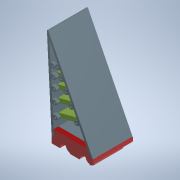
# Autodesk Inventor part: FingerEnclosure
Saved by Autodesk Inventor 2021 (Build 250183000, 183)
## iProperties
Created: 2020-03-10
Part Number: FingerEnclosure
Material: Generisch
Document SubType Name: Modeling
Designer: JochenAlt
Density: 1 g/cm^3
Appearance: Rot
Author: JochenAlt
Autodesk Inventor part; units mm, degrees
note: some values were not read from the file. Left out: dimensions or parameters whose unit could not be read.
ref_plane "YZ Plane" through (0, 0, 0) normal (1, 0, 0) x (0, 1, 0)
ref_plane "XZ Plane" through (0, 0, 0) normal (0, 1, 0) x (-1, 0, 0)
ref_plane "XY Plane" through (0, 0, 0) normal (0, 0, 1) x (1, 0, 0)
sketch "MainConstruction" plane through (0, 0, 0) normal (0, 0, 1) x (1, 0, 0)
  line L0 (-44.4573, 0) -> (45.9096, 0) construction
  line L1 (0, -41.3) -> (0, 41.3) construction
  line L2 (-12, 16.3923) -> (12, 16.3923) construction
  line L3 (6, -16.3923) -> (6, -10.3923) construction
  line L4 (6, -10.3923) -> (11.1962, -13.3923) construction
  line L5 (8.1962, -18.5885) -> (11.1962, -13.3923) construction
  line L6 (0, -16.3923) -> (6, -16.3923) construction
  line L7 (-6, -10.3923) -> (-6, -16.3923) construction
  line L8 (-6, -10.3923) -> (-11.1962, -13.3923) construction
  line L9 (0, 16.3923) -> (0, 0) construction
  line L10 (0, 0) -> (0, -16.3923) construction
  line L11 (-12, 14.3923) -> (12, 14.3923) construction
  line L12 (-12, 16.3923) -> (-12, 14.3923) construction
  line L13 (-12, 27) -> (12, 27) construction
  line L14 (-29.3827, -3.1077) -> (-17.3827, -23.8923) construction
  line L15 (0, 16.3923) -> (0, 27) construction
  line L16 (-23.3827, -13.5) -> (-14.1962, -8.1962) construction
  arc A0 (-2.6277, -14.0839) -> (-3.3698, -6.14) centre (-6, -10.3923) ccw construction
  arc A1 (3.3698, -6.14) -> (2.6277, -14.0839) centre (6, -10.3923) ccw construction
  line L17 (-27.2176, -1.8577) -> (-31.5477, -4.3577) construction
  line L18 (-15.2176, -22.6423) -> (-19.5477, -25.1423) construction
  line L19 (19.5477, -25.1423) -> (15.2176, -22.6423) construction
  circle A2 centre (0, 0) radius 22 construction
  line L20 (12, 14.3923) -> (12, 16.3923) construction
  line L21 (23.3827, -13.5) -> (14.1962, -8.1962) construction
  line L22 (20.1962, 2.1962) -> (14.1962, -8.1962) construction
  line L23 (11.1962, -13.3923) -> (14.1962, -8.1962) construction
  line L24 (-6, -16.3923) -> (0, -16.3923) construction
  line L25 (8.1962, -18.5885) -> (15.2176, -22.6423) construction
  line L26 (-15.2176, -22.6423) -> (-8.1962, -18.5885) construction
  line L27 (-12, 29.5) -> (-12, 24.5) construction
  line L28 (12, 29.5) -> (12, 24.5) construction
  line L29 (12, 24.5) -> (12, 16.3923) construction
  line L30 (-12, 24.5) -> (-12, 16.3923) construction
  line L31 (-11.1962, -13.3923) -> (-8.1962, -18.5885) construction
  line L32 (-11.1962, -13.3923) -> (-20.1962, 2.1962) construction
  line L33 (27.2176, -1.8577) -> (31.5477, -4.3577) construction
  line L34 (17.3827, -23.8923) -> (29.3827, -3.1077) construction
  line L35 (27.2176, -1.8577) -> (21.9687, 1.1728) construction
  line L36 (-27.2176, -1.8577) -> (-21.9687, 1.1728) construction
  line L37 (20.1962, 2.1962) -> (21.9687, 1.1728) construction
  line L38 (-21.9687, 1.1728) -> (-20.1962, 2.1962) construction
  line L39 (0, -16.3923) -> (0, -24.5) construction
  line L40 (0, -24.5) -> (0, -29.5) construction
  line L41 (0, -27) -> (24, -27) construction
  line L42 (18.4641, 3.1962) -> (6.4641, -17.5885) construction
  line L43 (-18.4641, 3.1962) -> (-6.4641, -17.5885) construction
  line L44 (-20.1962, 2.1962) -> (-18.4641, 3.1962) construction
  line L45 (20.1962, 2.1962) -> (18.4641, 3.1962) construction
  line L46 (3.3698, -6.14) -> (18.4641, 3.1962) construction
  line L47 (-18.4641, 3.1962) -> (-3.3698, -6.14) construction
  circle A3 centre (30.5, 27) radius 2.5 construction
  line L48 (12, 14.3923) -> (16.25, 14.3923) construction
  line L49 (16.25, 14.3923) -> (31.8962, 24.9262) construction
  line L50 (29.1038, 29.0738) -> (10.2677, 16.3923) construction
  line L51 (12, 16.3923) -> (10.2677, 16.3923) construction
  line L52 (8.1962, -18.5885) -> (6.4641, -17.5885) construction
  line L53 (6.4641, -17.5885) -> (2.6277, -14.0839) construction
  line L54 (-8.1962, -18.5885) -> (-6.4641, -17.5885) construction
  line L55 (-6.4641, -17.5885) -> (-2.6277, -14.0839) construction
sketch "Main" plane through (0, 0, 0) normal (0, 0, 1) x (1, 0, 0)
  line L0 (-20, 4) -> (-22.8714, 57.5994)
  line L1 (-23, 60) -> (-21.9249, 57.8498) construction
  line L2 (5, 4) -> (-20, 4)
  line L3 (-13.061, 37.1034) -> (-12.502, 35.9853)
  line L4 (-19.1427, 13.2337) -> (-18.7552, 6)
  line L5 (-19.7847, 25.2166) -> (-19.552, 20.8727) construction
  line L6 (-19.9203, 27.7479) -> (-19.6857, 23.3691)
  line L7 (-6.6518, 24.2849) -> (-4.3486, 19.6786)
  line L8 (-9.7309, 30.443) -> (-7.7698, 26.521)
  line L9 (-21.3047, 53.5907) -> (-16.1141, 43.2095)
  line L10 (-12.502, 35.9853) -> (-10.8489, 32.6791)
  line L11 (-21.3047, 53.5907) -> (-20.6838, 42.0008)
  line L12 (-20.2518, 33.9355) -> (-20.054, 30.2443)
  line L13 (-3.7896, 18.5606) -> (-3.2306, 17.4425)
  line L14 (-4.3486, 19.6786) -> (-3.7896, 18.5606)
  line L15 (-3.2306, 17.4425) -> (2.4907, 6) construction
  line L16 (-19.2765, 15.7301) -> (-19.7847, 25.2166) construction
  line L17 (-19.2096, 14.4819) -> (-19.2765, 15.7301)
  line L18 (-19.1427, 13.2337) -> (-19.2096, 14.4819)
  line L19 (-7.7698, 26.521) -> (-7.2108, 25.4029)
  line L20 (-7.2108, 25.4029) -> (-6.6518, 24.2849)
  line L21 (-6.6518, 24.2849) -> (-4.3486, 19.6786) construction
  line L22 (-19.7847, 25.2166) -> (-19.552, 20.8727)
  line L23 (-20.054, 30.2443) -> (-20.2518, 33.9355) construction
  line L24 (-19.9871, 28.9961) -> (-20.054, 30.2443)
  line L25 (-19.9203, 27.7479) -> (-19.9871, 28.9961)
  line L26 (-10.8489, 32.6791) -> (-10.2899, 31.5611)
  line L27 (-10.2899, 31.5611) -> (-9.7309, 30.443)
  line L28 (-9.7309, 30.443) -> (-7.7698, 26.521) construction
  line L29 (-20.3855, 36.4319) -> (-20.3186, 35.1837)
  line L30 (-13.6201, 38.2214) -> (-13.061, 37.1034)
  line L31 (-12.502, 35.9853) -> (-10.8489, 32.6791) construction
  line L32 (-20.2518, 33.9355) -> (-20.3186, 35.1837)
  line L33 (-18.7552, 6) -> (-19.1427, 13.2337) construction
  line L34 (-3.2306, 17.4425) -> (2.4907, 6)
  line L35 (-18.7552, 6) -> (2.4907, 6)
  arc A0 (-21.9249, 57.8498) -> (-22.8714, 57.5994) centre (-22.3721, 57.6262) ccw
  line L36 (-18.7552, 6) -> (-18.6481, 4)
  line L37 (2.4907, 6) -> (3.4907, 4)
  circle A1 centre (-12, 0) radius 1.05
  arc A2 (-14.9041, -0.7524) -> (-9, 0) centre (-12, 0) ccw
  circle A3 centre (0, 0) radius 1.05
  arc A4 (-3, 0) -> (3, 0) centre (0, 0) ccw
  line L38 (-9, 0) -> (-3, 0)
  arc A5 (3, 0) -> (5, 4) centre (2.5, 2.75) ccw
  line L39 (-18.7622, 8) -> (1.3789, 8)
  line L40 (-18.6551, 6) -> (-18.7622, 8)
  line L41 (1.3789, 8) -> (2.3789, 6)
  line L42 (-18.6604, 6.1) -> (2.3289, 6.1)
  arc A6 (3, 0) -> (-3, 0) centre (0, 0) ccw
  line L43 (2.1213, 2.1213) -> (3.9075, 0.3352)
  arc A7 (-9, 0) -> (-14.9041, -0.7524) centre (-12, 0) ccw
  line L44 (2.3789, 6) -> (3.3789, 4)
  line L45 (-18.6551, 6) -> (-18.5479, 4)
  line L46 (-20, 4) -> (-20, 0)
  line L47 (-21.9249, 57.8498) -> (5, 4)
  line L48 (-22.8714, 57.5994) -> (-23, 60) construction
  line L49 (-23, 60) -> (-23, 0) construction
  line L50 (0, -47.4) -> (0, 77.9) construction
  line L51 (-44.4573, 0) -> (45.9096, 0) construction
  line L52 (3, 0) -> (-23, 0) construction
  arc A8 (-14.9041, -0.7524) -> (-14.9041, -0.7524) centre (-12, 0) ccw
  line L53 (-15, 0) -> (-20, 0)
  line L54 (-15.2356, 0) -> (-14.7816, 1.1238)
  line L55 (-9.1468, 0.9271) -> (-8.8456, 0)
  line L56 (-8.8456, 0) -> (-9.1468, -0.9271)
  line L57 (-15.2356, 0) -> (-14.7816, -1.1238)
  line L58 (-2.7615, 1.1722) -> (-3.2591, 0)
  line L59 (-2.7615, -1.1722) -> (-3.2591, 0)
  line L60 (-20.3855, 36.4319) -> (-18.8876, 36.5122)
  arc A9 (-18.7539, 34.0157) -> (-18.8876, 36.5122) centre (-18.8208, 35.2639) ccw
  line L61 (-18.7539, 34.0157) -> (-20.2518, 33.9355)
  line L62 (-13.6201, 38.2214) -> (-14.9617, 37.5506)
  arc A10 (-14.9617, 37.5506) -> (-13.8437, 35.3145) centre (-14.4027, 36.4326) ccw
  line L63 (-13.8437, 35.3145) -> (-12.502, 35.9853)
  line L64 (-10.8489, 32.6791) -> (-12.1905, 32.0083)
  arc A11 (-12.1905, 32.0083) -> (-11.0725, 29.7722) centre (-11.6315, 30.8902) ccw
  line L65 (-11.0725, 29.7722) -> (-9.7309, 30.443)
  line L66 (-20.054, 30.2443) -> (-18.5562, 30.3245)
  arc A12 (-18.4224, 27.8281) -> (-18.5562, 30.3245) centre (-18.4893, 29.0763) ccw
  line L67 (-18.4224, 27.8281) -> (-19.9203, 27.7479)
  line L68 (-7.7698, 26.521) -> (-9.1115, 25.8501)
  arc A13 (-9.1115, 25.8501) -> (-7.9934, 23.6141) centre (-8.5525, 24.7321) ccw
  line L69 (-7.9934, 23.6141) -> (-6.6518, 24.2849)
  line L70 (-4.3486, 19.6786) -> (-5.6903, 19.0078)
  arc A14 (-5.6903, 19.0078) -> (-4.5723, 16.7717) centre (-5.1313, 17.8897) ccw
  line L71 (-4.5723, 16.7717) -> (-3.2306, 17.4425)
  line L72 (-19.2765, 15.7301) -> (-17.7786, 15.8103)
  arc A15 (-17.6449, 13.3139) -> (-17.7786, 15.8103) centre (-17.7117, 14.5621) ccw
  line L73 (-17.6449, 13.3139) -> (-19.1427, 13.2337)
  circle A16 centre (-14.4027, 36.4326) radius 0.5
  circle A17 centre (-18.8208, 35.2639) radius 0.5
  circle A18 centre (-18.4893, 29.0763) radius 0.5
  circle A19 centre (-11.6315, 30.8902) radius 0.5
  circle A20 centre (-8.5525, 24.7321) radius 0.5
  circle A21 centre (-17.7117, 14.5621) radius 0.5
  circle A22 centre (-5.1313, 17.8897) radius 0.5
  line L74 (-18.8208, 35.2639) -> (-14.4027, 36.4326) construction
  line L75 (-18.4893, 29.0763) -> (-11.6315, 30.8902) construction
  line L76 (-17.7117, 14.5621) -> (-5.1313, 17.8897) construction
  circle A23 centre (-19.3687, 40.8194) radius 0.5
  line L77 (-19.4356, 42.0677) -> (-20.6838, 42.0008)
  line L78 (-20.5501, 39.5044) -> (-19.3019, 39.5712)
  arc A24 (-19.3019, 39.5712) -> (-19.4356, 42.0677) centre (-19.3687, 40.8194) ccw
  line L79 (-20.5501, 39.5044) -> (-20.3855, 36.4319)
  line L80 (-20.6838, 42.0008) -> (-20.5501, 39.5044)
  circle A25 centre (-16.6731, 41.5325) radius 0.5
  arc A26 (-17.2321, 42.6505) -> (-16.1141, 40.4144) centre (-16.6731, 41.5325) ccw
  line L81 (-17.2321, 42.6505) -> (-16.1141, 43.2095)
  line L82 (-16.1141, 40.4144) -> (-14.9961, 40.9734)
  line L83 (-14.9961, 40.9734) -> (-13.6201, 38.2214)
  line L84 (-16.1141, 43.2095) -> (-14.9961, 40.9734)
  line L85 (-19.3687, 40.8194) -> (-16.6731, 41.5325) construction
  circle A27 centre (-18.121, 22.2012) radius 0.5
  line L86 (-18.1878, 23.4494) -> (-19.6857, 23.3691)
  line L87 (-18.0541, 20.953) -> (-19.552, 20.8727)
  line L88 (-19.552, 20.8727) -> (-19.2765, 15.7301)
  line L89 (-18.121, 22.2012) -> (-8.5525, 24.7321) construction
  line L90 (-18.7622, 8) -> (-18.8621, 7.9947)
  line L91 (1.3789, 8) -> (1.4907, 8)
  line L92 (-19.6857, 23.3691) -> (-19.552, 20.8727)
  line L93 (-18.121, 22.2012) -> (-19.6188, 22.1209) construction
  line L94 (-18.4893, 29.0763) -> (-20.159, 28.9869) construction
  line L95 (-18.8208, 35.2639) -> (-20.3186, 35.1837) construction
  line L96 (-19.3687, 40.8194) -> (-20.617, 40.7526) construction
  line L97 (-19.2096, 14.4819) -> (-17.7117, 14.5621) construction
  arc A28 (-18.0541, 20.953) -> (-18.1878, 23.4494) centre (-18.121, 22.2012) ccw
  line L98 (-18.949, 9.6168) -> (-10.2799, 11.9099) construction
  line L99 (-21.3047, 53.5907) -> (-10.2799, 11.9099) construction
  line L100 (-10.2799, 11.9099) -> (-1.6108, 14.2029) construction
  point P0 (-20.0171, 4.3184)
  point P1 (-18.5329, 1.8501)
  point P2 (0, 3)
  point P3 (-12, 3)
  point P4 (3.5032, 0.0324)
  point P5 (-16.5, 4)
  point P6 (-8.8456, 0)
  point P7 (-3.2591, 0)
  point P8 (-3.2591, 0)
  point P9 (-14.9041, -0.7524)
  point P10 (-18.8621, 7.9947)
  point P11 (2.9997, 0.0406)
  point P12 (-19.5609, 21.0395)
  dimension "d29" = 1.35
  dimension "d30" = 1.35
  dimension "d45" = 0.5
  dimension "d46" = 2
  dimension "d112" = 2.1
  dimension "d114" = 12
  dimension "d124" = 2
  dimension "d127" = 0.1
  dimension "d128" = 0.1
  dimension "d129" = 0.1
  dimension "d133" = 25
  dimension "d138" = 60
  dimension "d141" = 8.5
  dimension "d144" = 6.1965
  dimension "d145" = 8
  dimension "d147" = 68
  dimension "d148" = 135
  dimension "d149" = 72
  dimension "d150" = 67
  dimension "d151" = 3
  dimension "d152" = 4
  dimension "d154" = 3
  dimension "d155" = 1
  dimension "d156" = 1.25
  dimension "d176" = 7.65
  dimension "d177" = 6.885
  dimension "d178" = 5.5769
  dimension "d179" = 1.5
  constraints: 200 end point, 166 collinear, 45 point on circle, 41 tangent, 40 perpendicular, 32 point on line, 29 centre point, 22 equal radius, 21 coincident, 16 equal length, 6 horizontal, 6 parallel, 3 midpoint, 1 vertical, 9 other
  measures "d29" distance between parallel lines of L0 L11
  measures "d30" distance between parallel lines of L1 L9
  measures "d45" radius of A0
  measures "d46" distance between parallel lines of L2 L35
  measures "d112" diameter of A1
  measures "d114" distance of A3.centre A1.centre
  measures "d124" distance between parallel lines of L39 L35
  measures "d127" distance between parallel lines of L40 L4
  measures "d128" distance between parallel lines of L34 L41
  measures "d129" distance between parallel lines of L42 L35
  measures "d133" distance of L2.start L0.start
  measures "d138" distance of L1.start L49.end
  measures "d141" distance of L17.start L40.start
  measures "d144" distance of L32.end L24.start
  measures "d145" distance from line of A7.centre L46
  measures "d147" angle of L53 L54
  measures "d148" angle of L51 L43
  measures "d149" angle of L38 L55
  measures "d150" angle of L38 L58
  measures "d151" radius of A2
  measures "d152" distance between parallel lines of L2 L52
  measures "d154" distance of L46.end L49.end
  measures "d155" diameter of A16
  measures "d156" radius of A10
  measures "d176" distance of L17.start L93.end
  measures "d177" distance of L93.end L24.start
  measures "d178" distance of L32.end L96.end
  measures "d179" distance of L29.start L60.end
extrude "Extrusion1" add sketch "Main" along normal mid plane 18 contours L0 A0 L47 L2 L37 L34 L13 L14 L7 L20 L19 L8 L27 L26 L10 L3 L30 L83 L84 L9 L11 L80 L79 L29 L32 L12 L24 L25 L6 L22 L88 L17 L18 L4 L36 | L36 L35 L45 L2 | L45 L35 L44 L2 | L4 L90 L40 L35 | L44 L35 L37 L2 | L40 L42 L41 L35 | L41 L91 L34 L35 | L40 L39 L41 L42 | L18 L17 L72 A15 L73 | L71 A14 L70 L14 L13 | L22 L86 A28 L87 | L69 A13 L68 L19 L20 | L25 L24 L66 A12 L67 | L65 A11 L64 L26 L27 | L32 L29 L60 A9 L61 | L63 A10 L62 L30 L3 | L80 L77 A24 L78 | L82 A26 L81 L84
extrude "Extrusion16" add sketch "Main" along normal mid plane 24 contours L0 A0 L47 L2 L37 L34 L13 L14 L7 L20 L19 L8 L27 L26 L10 L3 L30 L83 L84 L9 L11 L80 L79 L29 L32 L12 L24 L25 L6 L22 L88 L17 L18 L4 L36 | L18 L17 L72 A15 L73 | L71 A14 L70 L14 L13 | L22 L86 A28 L87 | L69 A13 L68 L19 L20 | L25 L24 L66 A12 L67 | L65 A11 L64 L26 L27 | L32 L29 L60 A9 L61 | L63 A10 L62 L30 L3 | L80 L77 A24 L78 | L82 A26 L81 L84
extrude "Extrusion22" cut sketch "Main" against normal mid plane 20 contours L18 L17 L72 A15 L73 | L71 A14 L70 L14 L13 | L22 L86 A28 L87 | L69 A13 L68 L19 L20 | L25 L24 L66 A12 L67 | L65 A11 L64 L26 L27 | L32 L29 L60 A9 L61 | L63 A10 L62 L30 L3 | L80 L77 A24 L78 | L82 A26 L81 L84
extrude "Extrusion17" add sketch "Main" along normal mid plane 17 separate body contours L2 A5 L43 A6 L58 L38 L55 A7 L54 L53 L46 | L54 A7 L53 | A7 A2 | A5 A6 L43 | L55 L38 A7 | A2 L38 L56 | A4 A6 | L59 L38 A4 | A6 L38 L58
extrude "Extrusion18" add sketch "Main" along normal mid plane 24 contours L2 A5 L43 A6 L58 L38 L55 A7 L54 L53 L46 | L45 L35 L44 L2 | L54 A7 L53 | L40 L42 L41 L35 | A5 A6 L43 | L40 L39 L41 L42 bodies 2
extrude "Extrusion19" cut sketch "Main" along normal mid plane 20.25 contours L36 L35 L45 L2 | L45 L35 L44 L2 | L44 L35 L37 L2 | L40 L42 L41 L35 bodies 2
extrude "Extrusion20" cut sketch "Main" along normal mid plane 18 contours L40 L42 L41 L35 | L40 L39 L41 L42 bodies 2
sketch "rig" plane through (0, 0, 0) normal (0, 0, 1) x (1, 0, 0)
  circle A0 centre (-18.8208, 35.2639) radius 0.5 projected
  circle A1 centre (-19.3687, 40.8194) radius 0.5 projected
  circle A2 centre (-16.6731, 41.5325) radius 0.5 projected
  circle A3 centre (-14.4027, 36.4326) radius 0.5 projected
  circle A4 centre (-11.6315, 30.8902) radius 0.5 projected
  circle A5 centre (-8.5525, 24.7321) radius 0.5 projected
  circle A6 centre (-18.121, 22.2012) radius 0.5 projected
  circle A7 centre (-17.7117, 14.5621) radius 0.5 projected
  circle A8 centre (-5.1313, 17.8897) radius 0.5 projected
  line L0 (-18.0314, 15.7706) -> (-5.4509, 19.0982)
  arc A9 (-4.8116, 16.6813) -> (-5.4509, 19.0982) centre (-5.1313, 17.8897) ccw
  line L1 (-4.8116, 16.6813) -> (-17.3921, 13.3537)
  arc A10 (-18.0314, 15.7706) -> (-17.3921, 13.3537) centre (-17.7117, 14.5621) ccw
  line L2 (-18.4406, 23.4096) -> (-8.8721, 25.9406)
  line L3 (-17.8013, 20.9927) -> (-8.2328, 23.5237)
  arc A11 (-18.4406, 23.4096) -> (-17.8013, 20.9927) centre (-18.121, 22.2012) ccw
  arc A12 (-8.2328, 23.5237) -> (-8.8721, 25.9406) centre (-8.5525, 24.7321) ccw
  line L4 (-18.8089, 30.2848) -> (-11.9512, 32.0987)
  line L5 (-18.1696, 27.8679) -> (-11.3119, 29.6818)
  arc A13 (-18.8089, 30.2848) -> (-18.1696, 27.8679) centre (-18.4893, 29.0763) ccw
  arc A14 (-11.3119, 29.6818) -> (-11.9512, 32.0987) centre (-11.6315, 30.8902) ccw
  circle A15 centre (-18.4893, 29.0763) radius 0.5 projected
  line L6 (-18.5011, 34.0555) -> (-14.083, 35.2241)
  arc A16 (-14.083, 35.2241) -> (-14.7223, 37.641) centre (-14.4027, 36.4326) ccw
  line L7 (-14.7223, 37.641) -> (-19.1404, 36.4724)
  arc A17 (-19.1404, 36.4724) -> (-18.5011, 34.0555) centre (-18.8208, 35.2639) ccw
  arc A18 (-19.6884, 42.0279) -> (-19.0491, 39.611) centre (-19.3687, 40.8194) ccw
  arc A19 (-16.3535, 40.324) -> (-16.9928, 42.7409) centre (-16.6731, 41.5325) ccw
  line L8 (-19.6884, 42.0279) -> (-16.9928, 42.7409)
  line L9 (-19.0491, 39.611) -> (-16.3535, 40.324)
  point P0 (0, 0)
  dimension "d173" = 2.5
  constraints: 21 end point, 20 point on circle, 20 tangent, 10 centre point, 10 coincident, 5 equal radius, 4 parallel
  measures "d173" distance between parallel lines of L1 L0
extrude "Extrusion23" add sketch "rig" along normal mid plane 19 separate body
equation "\"d30\" = d29"
equation "\"d5\" = d20"
equation "\"roundness_small\" = 3"
equation "\"roundness_tiny\" = 0.5"
equation "\"wall_thickness\" = 3"
equation "\"medium_arm_width\" = 51"
equation "\"big_arm_width\" = 56"
equation "\"medium_arm_radius\" = 35"
equation "\"big_arm_radius\" = 48"
equation "\"medium_arm_circle_centre\" = 11"
equation "\"big_arm_circle_centre\" = 25"
equation "\"thickness\" = 3"
equation "\"tight_fit\" = 0.2"
equation "\"press_fit\" = 0.1"
equation "\"m2_screw_hole_diameter\" = 2.2"
equation "\"m2_hex_width\" = 4.2"
equation "\"m2_washer_diameter\" = 5.2"
equation "\"m2_allen_screw_width\" = 4"
equation "\"m2_allen_screw_height\" = 2"
equation "\"m2_washer_height\" = 0.3"
equation "\"d20\" = 1"
